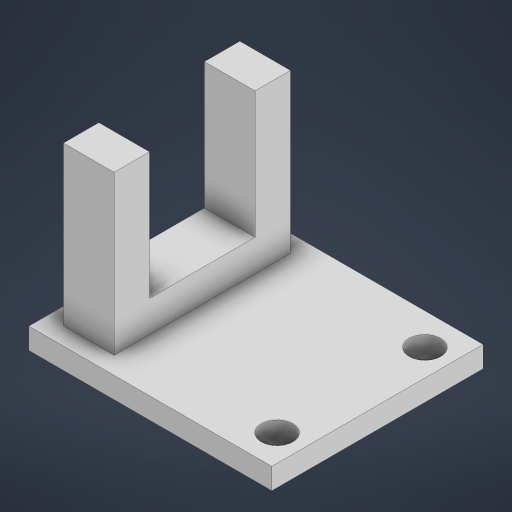
# Autodesk Inventor part: lichtschrankenmodulmodell
Saved by Autodesk Inventor 2024 (Build 280153000, 153)
## iProperties
Created: 2026-03-30
Part Number: lichtschrankenmodulmodell
Material: Generic
Document SubType Name: Modeling
Designer: schar
Density: 1 g/cm^3
Appearance: Default
Author: schar
Autodesk Inventor part; units mm, degrees
ref_plane "YZ Plane" through (0, 0, 0) normal (1, 0, 0) x (0, 1, 0)
ref_plane "XZ Plane" through (0, 0, 0) normal (0, 1, 0) x (-1, 0, 0)
ref_plane "XY Plane" through (0, 0, 0) normal (0, 0, 1) x (1, 0, 0)
sketch "Sketch1" plane through (0, 0, 0) normal (0, 1, 0) x (-1, 0, 0)
  line L0 (11.5, 10) -> (-11.5, 10)
  line L1 (-11.5, 10) -> (-11.5, -10)
  line L2 (-11.5, -10) -> (11.5, -10)
  line L3 (11.5, -10) -> (11.5, 10)
  line L4 (11.5, 10) -> (-11.5, -10) construction
  line L5 (-11.5, 10) -> (11.5, -10) construction
  line L6 (-11.5, 0) -> (-11.5, -7)
  line L7 (-11.5, 0) -> (-11.5, 7)
  line L8 (-11.5, 7) -> (-9, 7)
  circle A0 centre (-9, 7) radius 1.5
  line L9 (-11.5, -7) -> (-9, -7)
  circle A1 centre (-9, -7) radius 1.5
  point P0 (0, 0)
  dimension "d0" = 23
  dimension "d1" = 20
  dimension "d2" = 7
  dimension "d3" = 7
  dimension "d4" = 2.5
  dimension "d5" = 3
  dimension "d6" = 3
  constraints: 20 end point, 3 horizontal, 3 midpoint, 2 centre point, 2 coincident, 2 parallel, 2 point on line, 1 perpendicular
  measures "d0" distance of L2.end L1.end
  measures "d1" distance of L1.end L0.end
  measures "d2" distance of L6.start L6.end
  measures "d3" distance of L6.start L7.end
  measures "d4" distance of L7.end L8.end
  measures "d5" diameter of A0
  measures "d6" diameter of A1
extrude "Extrusion1" add sketch "Sketch1" along normal blind 2
sketch "Sketch2" plane through (0, 2, 0) normal (0, 1, 0) x (1, 0, 0)
  line L0 (-5.0848, -8.3507) -> (-9.8803, -8.3507)
  line L1 (-9.8803, -8.3507) -> (-9.8803, 8.3507)
  line L2 (-9.8803, 8.3507) -> (-5.0848, 8.3507)
  line L3 (-5.0848, 8.3507) -> (-5.0848, -8.3507)
  line L4 (-5.0848, -8.3507) -> (-9.8803, 8.3507) construction
  line L5 (-9.8803, -8.3507) -> (-5.0848, 8.3507) construction
  line L6 (-9.8803, 0) -> (-9.8803, 5)
  line L7 (-9.8803, 0) -> (-9.8803, -5)
  line L8 (-9.8803, -5) -> (-5.0848, -5)
  line L9 (-5.0848, -5) -> (-5.0848, -8.3507)
  line L10 (-5.0848, -8.3507) -> (-9.8803, -8.3507)
  line L11 (-9.8803, -8.3507) -> (-9.8803, -5)
  line L12 (-9.8803, 5) -> (-5.0848, 5)
  line L13 (-5.0848, 5) -> (-5.0848, 8.3507)
  line L14 (-5.0848, 8.3507) -> (-9.8803, 8.3507)
  line L15 (-9.8803, 8.3507) -> (-9.8803, 5)
  point P0 (0, 0)
  point P1 (-7.4826, 0)
  dimension "d9" = 5
  dimension "d10" = 5
  constraints: 32 end point, 6 parallel, 3 horizontal, 3 midpoint, 3 perpendicular, 2 point on line
  measures "d9" distance of L6.start L6.end
  measures "d10" distance of L6.start L7.end
extrude "Extrusion2" add sketch "Sketch2" along normal blind 15 contours L0 L1 L8 L3 | L12 L1 L2 L3
sketch "Sketch3" plane through (0, 2, 0) normal (0, 1, 0) x (1, 0, 0)
  line L0 (-5.0848, -8.3507) -> (-5.0848, -5) projected
  line L1 (-9.8803, 5) -> (-5.0848, 5) projected
  line L2 (-5.0848, -5) -> (-9.8803, -5)
  line L3 (-9.8803, -5) -> (-9.8803, 5)
  line L4 (-9.8803, 5) -> (-5.0848, 5)
  line L5 (-5.0848, 5) -> (-5.0848, -5)
  point P0 (0, 0)
  constraints: 8 end point, 2 parallel, 1 horizontal, 1 perpendicular
extrude "Extrusion3" add sketch "Sketch3" along normal blind 3
body "Solid1"
